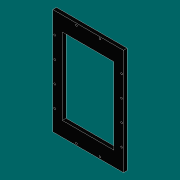
# Autodesk Inventor part: front
Saved by Autodesk Inventor 2016 (Build 200138000, 138)
## iProperties
Created: 2015-10-05
Part Number: front
Material: ABS Plastic
Document SubType Name: Modeling
Designer: Sawaiz
Density: 1.06 g/cm^3
Appearance: Smooth - Black
Author: Sawaiz
Autodesk Inventor part; units mm, degrees
ref_plane "YZ Plane" through (0, 0, 0) normal (1, 0, 0) x (0, 1, 0)
ref_plane "XZ Plane" through (0, 0, 0) normal (0, 1, 0) x (-1, 0, 0)
ref_plane "XY Plane" through (0, 0, 0) normal (0, 0, 1) x (1, 0, 0)
sketch "Sketch1" plane through (0, 0, 0) normal (0, 1, 0) x (-1, 0, 0)
  line L0 (60, -90) -> (-60, -90)
  line L1 (-60, -90) -> (-60, 90)
  line L2 (-60, 90) -> (60, 90)
  line L3 (60, 90) -> (60, -90)
  line L4 (60, -90) -> (-60, 90) construction
  line L5 (-60, -90) -> (60, 90) construction
  point P0 (0, 0)
  dimension "d0" = 120
  dimension "d1" = 180
  constraints: 12 end point, 2 midpoint, 2 parallel, 1 horizontal, 1 perpendicular
  measures "d0" distance of L1.end L2.end
  measures "d1" distance of L0.end L1.end
extrude "Extrusion1" add sketch "Sketch1" along normal blind 6.35
sketch "Sketch2" plane through (0, 0, 0) normal (0, -1, 0) x (1, 0, 0)
  line L0 (-43.8, -65) -> (43.8, -65)
  line L1 (43.8, -65) -> (43.8, 65)
  line L2 (43.8, 65) -> (-43.8, 65)
  line L3 (-43.8, 65) -> (-43.8, -65)
  line L4 (-43.8, -65) -> (43.8, 65) construction
  line L5 (43.8, -65) -> (-43.8, 65) construction
  line L6 (60, 90) -> (-60, 90) projected
  point P0 (0, 0)
  dimension "d4" = 87.6
  dimension "d8" = 25
  constraints: 12 end point, 2 midpoint, 2 parallel, 1 horizontal, 1 perpendicular
  measures "d4" distance of L2.end L1.end
  measures "d8" distance between parallel lines of L6 L2
extrude "Extrusion2" cut sketch "Sketch2" against normal through all
sketch "Sketch3" plane through (0, 0, 0) normal (0, -1, 0) x (1, 0, 0)
  line L0 (43.8, 65) -> (43.8, -65) projected
  line L1 (43.8, -65) -> (-43.8, -65) projected
  line L2 (-43.8, -65) -> (-43.8, 65) projected
  line L3 (-43.8, 65) -> (43.8, 65) projected
  line L4 (-60, -90) -> (60, -90) projected
  line L5 (60, -90) -> (60, 90) projected
  line L6 (60, 90) -> (-60, 90) projected
  line L7 (-60, 90) -> (-60, -90) projected
  line L8 (56.825, 54) -> (56.825, 18)
  line L9 (56.825, 18) -> (-56.825, 18)
  line L10 (-56.825, 18) -> (-56.825, 54)
  line L11 (-20, 86.825) -> (-20, -86.825)
  line L12 (-20, -86.825) -> (20, -86.825)
  line L13 (-43.8, 65) -> (-43.8, -65) projected
  line L14 (20, -86.825) -> (20, 86.825)
  line L15 (56.825, -54) -> (56.825, -18)
  line L16 (56.825, -18) -> (-56.825, -18)
  line L17 (-43.8, 65) -> (43.8, 65) projected
  line L18 (43.8, -65) -> (-43.8, -65) projected
  line L19 (-56.825, -18) -> (-56.825, 18)
  line L20 (-56.825, -54) -> (-56.825, -18)
  line L21 (56.825, -18) -> (56.825, 18)
  line L22 (-56.825, -54) -> (56.825, -54)
  line L23 (-56.825, 54) -> (56.825, 54)
  line L24 (-20, 86.825) -> (20, 86.825)
  point P0 (0, 0)
  dimension "d9" = 3.175
  dimension "d10" = 3.175
  dimension "d11" = 3.175
  dimension "d12" = 3.175
  dimension "d20" = 40
  dimension "d21" = 40
  dimension "d22" = 36
  dimension "d24" = 36
  constraints: 29 end point, 5 vertical, 3 collinear, 3 horizontal, 3 parallel, 2 perpendicular
  measures "d9" distance between parallel lines of L7 L10
  measures "d10" distance from line of L5 L8.start
  measures "d11" distance from line of L6 L14.end
  measures "d12" distance between parallel lines of L4 L12
  measures "d20" distance from line of L7 L11.start
  measures "d21" distance of L11.start L14.end
  measures "d22" distance from line of L4 L20.start
  measures "d24" distance of L20.start L16.end
hole "Hole1" at (-20, 0, 86.825) at (20, 0, 86.825) at (56.825, 0, 54) at (56.825, 0, 18) at (56.825, 0, -54) at (20, 0, -86.825) at (-20, 0, -86.825) at (-56.825, 0, -54) at (-56.825, 0, -18) at (-56.825, 0, 18) at (-56.825, 0, 54) at (56.825, 0, -18) direction (0, 1, 0) diameter 3 end through all
equation "\"d0\" = width"
equation "\"d1\" = height"
equation "\"d2\" = materialThickness"
equation "\"d4\" = cardWidth + 4 * cardClearence"
equation "\"d6\" = materialThickness"
equation "\"d9\" = 0.5 * materialThickness"
equation "\"d10\" = 0.5 * materialThickness"
equation "\"d11\" = 0.5 * materialThickness"
equation "\"d12\" = 0.5 * materialThickness"
equation "\"d20\" = 0.333333 * width"
equation "\"d21\" = 0.333333 * width"
equation "\"d22\" = 0.2 * height"
equation "\"d24\" = 0.2 * height"
equation "\"height\" = 180"
equation "\"width\" = 120"
equation "\"depth\" = 115"
equation "\"materialThickness\" = 6.35"
equation "\"laserKerf\" = 0.1"
equation "\"cardPinDiameter\" = 3"
equation "\"spoolDiameter\" = 95"
equation "\"cardThickness\" = 0.76"
equation "\"cardFillet\" = 2.88"
equation "\"cardHeight\" = 53.98"
equation "\"cardSelected\" = 1"
equation "\"cardWidth\" = 85.6"
equation "\"centeralShaftDiameter\" = 8"
equation "\"cardClearence\" = 0.5"
equation "\"bearingOd\" = 22"
equation "\"bearingWidth\" = 8"
equation "\"axleHeight\" = 95"
equation "\"nutTrapClearence\" = 2"
equation "\"nutTrapwidth\" = 5.5"
equation "\"nutTrapDepth\" = 2.5"
body "Solid1"
